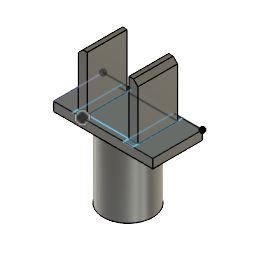
Grabber hand (Autodesk Fusion 360 design; units mm, degrees)
part number: 2026-03-29-09-07-12-309
Autodesk Fusion 360 part; units mm, degrees
note: some values were not read from the file. Set by a fixed rule: which sketch regions a step uses.
sketch "Sketch1" plane through (0, 0, 0) normal (0, 0, 1) x (1, 0, 0)
  circle A0 centre (0, 0) radius 27.5
  dimension "d1" = 55
  constraint coincident A0.centre origin
  measures "d1" diameter of A0
extrude "Extrude1" add sketch "Sketch1" along normal blind 74
sketch "Sketch2" plane through (0, 0, 74) normal (0, 0, 1) x (-1, 0, 0)
  circle A0 centre (0, 0) radius 27.5
  line L0 (0, -27.5) -> (-55, -27.5)
  line L1 (-55, -27.5) -> (-55, 27.5)
  line L2 (-55, 27.5) -> (0, 27.5)
  line L3 (0, -27.5) -> (55, -27.5)
  line L4 (0, 27.5) -> (55, 27.5)
  line L5 (55, -27.5) -> (55, 27.5)
  dimension "d4" = 55
  dimension "d14" = 55
  constraint coincident A0 L0.start
  constraint coincident A0 L2.end
  constraint tangent A0 L0
  constraint perpendicular L0 L1
  constraint tangent A0 L2
  constraint tangent A0 L3
  constraint tangent A0 L4
  constraint vertical L5
  constraint coincident L4 L5.end
  constraint perpendicular L4 L5
  measures "d4" distance of L0.start L3.end
  measures "d14" distance of L2.end L4.end
extrude "Extrude2" add sketch "Sketch2" along normal blind 10
sketch "Sketch3" plane through (0, 0, 84) normal (0, 0, 1) x (-1, 0, 0)
  line L0 (-55, -27.5) -> (55, -27.5)
  line L1 (55, 27.5) -> (-55, 27.5)
  line L2 (-55, 27.5) -> (-55, -27.5)
  line L3 (55, -27.5) -> (33, -27.5)
  line L4 (33, -27.5) -> (23, -27.5)
  line L5 (-55, -27.5) -> (-33, -27.5)
  line L6 (-33, -27.5) -> (-23, -27.5)
  line L7 (-23, -27.5) -> (-23, 27.5)
  line L8 (-23, 27.5) -> (-33, 27.5)
  line L9 (-33, 27.5) -> (-33, -27.5)
  line L10 (55, -27.5) -> (55, 27.5)
  line L11 (33, -27.5) -> (33, -22)
  line L12 (33, -22) -> (23, -22)
  line L13 (23, -22) -> (23, -27.5)
  line L14 (33, -22) -> (33, 27.5)
  line L15 (23, -22) -> (23, 27.5)
  line L16 (33, 27.5) -> (33, 22)
  line L17 (33, 22) -> (23, 22)
  line L18 (23, -22) -> (-33, -22)
  line L19 (23, 22) -> (-33, 22)
  dimension "d8" = 10
  dimension "d10" = 10
  dimension "d15" = 5.5
  dimension "d16" = 5.5
  constraint coincident L0.end L3.start
  constraint perpendicular L2 L3
  constraint horizontal L4
  constraint coincident L0.start L2.end
  constraint perpendicular L2 L5
  constraint horizontal L6
  constraint vertical L7
  constraint horizontal L8
  constraint vertical L9
  constraint vertical L11
  constraint perpendicular L11 L12
  constraint perpendicular L1 L14
  constraint coincident L1 L15.end
  constraint perpendicular L1 L15
  constraint perpendicular L1 L16
  constraint coincident L15 L17.end
  constraint perpendicular L15 L17
  constraint coincident L9 L18.end
  constraint perpendicular L9 L18
  constraint horizontal L19
  constraint coincident L9 L19.end
  measures "d8" distance of L3.end L4.end
  measures "d10" distance of L5.end L6.end
  measures "d15" distance of L3.end L11.end
  measures "d16" distance of L14.end L16.end
extrude "Extrude4" add sketch "Sketch3" along normal blind 60 contours L7 L9 L18 L19 | L12 L14 L15 L17
chamfer "Chamfer2" distance 5 angle 45 1 edges at (-33, 0, 144)
chamfer "Chamfer3" distance 5 angle 45 1 edges at (33, 0, 144)
sketch "Sketch5" plane through (0, 0, 0) normal (0, 1, 0) x (1, 0, 0)
equation "d15 = ( 55 / 10 ) * 1 mm"
equation "d16 = ( 55 / 10 ) * 1 mm"
